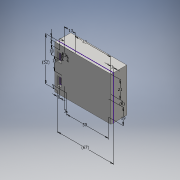
# Autodesk Inventor part: Bund
Saved by Autodesk Inventor 2016 (Build 200138000, 138)
## iProperties
Created: 2016-12-11
Part Number: Bund
Material: Generic
Document SubType Name: Modeling
Designer: Simon
Density: 1 g/cm^3
Appearance: Default
Author: Simon
Autodesk Inventor part; units mm, degrees
ref_plane "YZ Plane" through (0, 0, 0) normal (1, 0, 0) x (0, 1, 0)
ref_plane "XZ Plane" through (0, 0, 0) normal (0, 1, 0) x (-1, 0, 0)
ref_plane "XY Plane" through (0, 0, 0) normal (0, 0, 1) x (1, 0, 0)
sketch "Sketch1" plane through (0, 0, 0) normal (0, 1, 0) x (-1, 0, 0)
  line L0 (-33.5, 26) -> (33.5, 26)
  line L1 (33.5, 26) -> (33.5, -26)
  line L2 (-33.5, -26) -> (-33.5, 26)
  line L3 (-33.5, 26) -> (33.5, -26) construction
  line L4 (33.5, 26) -> (-33.5, -26) construction
  line L5 (33.5, 0) -> (28, 0)
  line L6 (28, 7.5) -> (28, -7.5)
  line L7 (30.5, 7.5) -> (25.5, 7.5)
  line L8 (25.5, 7.5) -> (25.5, 17.5)
  line L9 (25.5, 17.5) -> (30.5, 17.5)
  line L10 (30.5, 17.5) -> (30.5, 7.5)
  line L11 (30.5, -7.5) -> (25.5, -7.5)
  line L12 (25.5, -7.5) -> (25.5, -17.5)
  line L13 (25.5, -17.5) -> (30.5, -17.5)
  line L14 (30.5, -17.5) -> (30.5, -7.5)
  line L15 (22.5, -23) -> (-27.5, -23)
  line L16 (-27.5, -23) -> (-27.5, -4)
  line L17 (-27.5, -4) -> (22.5, -4)
  line L18 (22.5, -4) -> (22.5, -23)
  line L19 (12.5, 23) -> (-30.5, 23)
  line L20 (-30.5, 23) -> (-30.5, 2)
  line L21 (-30.5, 2) -> (12.5, 2)
  line L22 (12.5, 2) -> (12.5, 23)
  line L23 (25.5, 12.5) -> (12.5, 12.5)
  line L24 (-33.5, -26) -> (33.5, -26)
  line L25 (12.5, 16.5) -> (25.5, 16.5)
  line L26 (12.5, 8.5) -> (25.5, 8.5)
  line L27 (25.5, 16.5) -> (22.5, 16.5)
  line L28 (22.5, 16.5) -> (22.5, 13.5)
  line L29 (22.5, 13.5) -> (25.5, 13.5)
  line L30 (22.5, 13.5) -> (22.5, 11.5)
  line L31 (22.5, 11.5) -> (22.5, 8.5)
  line L32 (22.5, 11.5) -> (25.5, 11.5)
  line L33 (24.2677, 11.5) -> (24.2677, 13.5)
  point P0 (0, 0)
  point P1 (24.2677, 12.5)
  dimension "d3" = 15
  dimension "d5" = 10
  dimension "d6" = 5
  dimension "d11" = 50
  dimension "d12" = 3
  dimension "d13" = 43
  dimension "d14" = 13
  dimension "d22" = 19
  dimension "d23" = 21
  dimension "d26" = 3
  dimension "d27" = 3
  dimension "d28" = 3
  dimension "d29" = 3
  dimension "d30" = 6
  dimension "d31" = 67
  dimension "d32" = 52
  dimension "d33" = 8
  dimension "d34" = 3
  dimension "d35" = 2
  constraints: 68 end point, 13 point on line, 11 perpendicular, 9 midpoint, 9 parallel, 8 horizontal, 2 equal length, 1 vertical
  measures "d3" distance of L6.start L6.end
  measures "d5" distance of L9.end L7.start
  measures "d6" distance of L8.end L9.end
  measures "d11" distance of L15.start L15.end
  measures "d12" distance between parallel lines of L12 L18
  measures "d13" distance of L19.start L19.end
  measures "d14" distance between parallel lines of L22 L8
  measures "d22" distance of L15.end L16.end
  measures "d23" distance of L19.end L20.end
  measures "d26" distance between parallel lines of L24 L15
  measures "d27" distance between parallel lines of L20 L2
  measures "d28" distance between parallel lines of L1 L14
  measures "d29" distance between parallel lines of L0 L19
  measures "d30" distance between parallel lines of L17 L21
  measures "d31" distance between parallel lines of L2 L1
  measures "d32" distance between parallel lines of L24 L0
  measures "d33" distance between parallel lines of L25 L26
  measures "d34" distance of L25.end L27.end
  measures "d35" distance of L28.end L30.end
extrude "Extrusion1" add sketch "Sketch1" along normal blind 16 contours L0 L1 L24 L2 | L26 L31 L32 L8 | L32 L33 L23 L8 | L26 L22 L23 L30 L31 | L8 L29 L28 L25 | L23 L33 L29 L8 | L32 L30 L23 L33 | L28 L30 L23 L22 L25 | L23 L30 L29 L33
sketch "Sketch2" plane through (0, 16, 0) normal (0, 1, 0) x (1, 0, 0)
  line L0 (-12.5, -16.5) -> (-25.5, -16.5) projected
  line L1 (-12.5, -8.5) -> (-25.5, -8.5) projected
  line L2 (-22.5, -11.5) -> (-22.5, -8.5) projected
  line L3 (-22.5, -16.5) -> (-22.5, -13.5) projected
  line L4 (-22.5, -11.5) -> (-25.5, -11.5) projected
  line L5 (-22.5, -13.5) -> (-25.5, -13.5) projected
  line L6 (-25.5, -7.5) -> (-25.5, -17.5) projected
  line L7 (-12.5, -2) -> (-12.5, -23) projected
  line L8 (-22.5, -13.5) -> (-22.5, -11.5) projected
  point P0 (0, 0)
extrude "Extrusion4" cut sketch "Sketch2" against normal blind 13 contours L0 L3 L8 L2 L1 L7
extrude "Extrusion5" cut sketch "Sketch2" against normal blind 10 contours L5 L6 L4 L8
extrude "Extrusion6" add sketch "Sketch1" against normal blind 3 contours L0 L1 L24 L2 | L26 L31 L32 L8 | L32 L33 L23 L8 | L26 L22 L23 L30 L31 | L8 L29 L28 L25 | L23 L33 L29 L8 | L32 L30 L23 L33 | L22 L21 L20 L19 | L28 L30 L23 L22 L25 | L23 L30 L29 L33 | L15 L16 L17 L18
body "Solid1"
